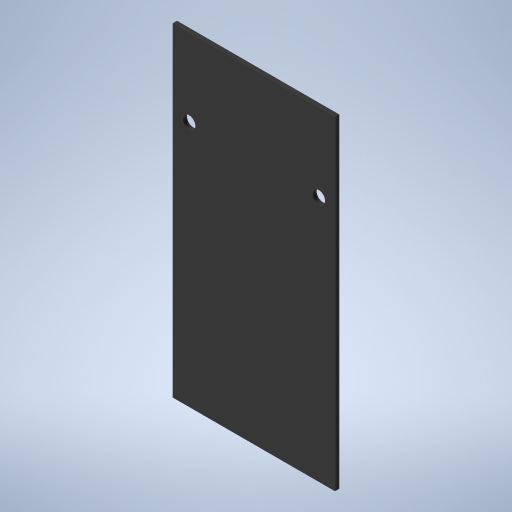
# Autodesk Inventor part: Kicker Poly Top Part
Saved by Autodesk Inventor 2023 (Build 270158000, 158)
## iProperties
Created: 2024-03-11
Part Number: Kicker Poly Top Part
Material: Generic
Document SubType Name: Modeling
Designer: Robodox
Density: 1 g/cm^3
Appearance: Default
Author: Robodox
Autodesk Inventor part; units mm, degrees
ref_plane "YZ Plane" through (0, 0, 0) normal (1, 0, 0) x (0, 1, 0)
ref_plane "XZ Plane" through (0, 0, 0) normal (0, 1, 0) x (-1, 0, 0)
ref_plane "XY Plane" through (0, 0, 0) normal (0, 0, 1) x (1, 0, 0)
sketch "Sketch1" plane through (0, 0, 0) normal (0, 0, 1) x (1, 0, 0)
  line L0 (-39.8758, 37.0237) -> (23.6242, 37.0237)
  line L1 (23.6242, 37.0237) -> (23.6242, -89.9763)
  line L2 (23.6242, -89.9763) -> (-39.8758, -89.9763)
  line L3 (-39.8758, -89.9763) -> (-39.8758, 37.0237)
  line L4 (23.6242, 37.0237) -> (23.6242, 6.5437)
  line L5 (23.6242, 6.5437) -> (17.2742, 6.5437)
  circle A0 centre (17.2742, 6.5437) radius 2.54
  line L6 (17.2742, 6.5437) -> (-33.5258, 6.5437)
  circle A1 centre (-33.5258, 6.5437) radius 2.54
  point P0 (0, 0)
  dimension "d0" = 63.5
  dimension "d1" = 127
  dimension "d4" = 30.48
  dimension "d5" = 6.35
  dimension "d6" = 5.08
  dimension "d7" = 50.8
  dimension "d8" = 5.08
  constraints: 14 end point, 2 centre point, 2 coincident, 2 horizontal, 2 parallel, 2 perpendicular, 1 point on line
  measures "d0" distance of L0.start L0.end
  measures "d1" distance of L2.end L0.start
  measures "d4" distance of L0.end L4.end
  measures "d5" distance of L4.end L5.end
  measures "d6" diameter of A0
  measures "d7" distance of L6.start L6.end
  measures "d8" diameter of A1
extrude "Extrusion2" add sketch "Sketch1" along normal blind 1.5875
body "Solid2"
